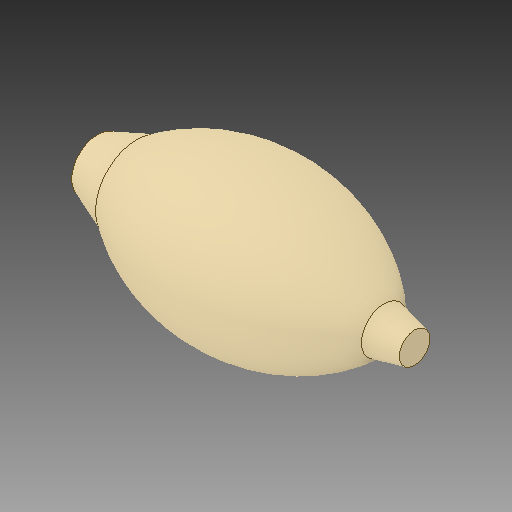
# Autodesk Inventor part: Armbu
Saved by Autodesk Inventor 2019 (Build 230136000, 136)
## iProperties
Created: 2020-04-02
Part Number: Armbu
Material: Generic
Document SubType Name: Modeling
Designer: Jurgen
Density: 1 g/cm^3
Appearance: Beige
Mass: 1875.66 g
Surface Area: 804.648 cm^2
Volume: 1875.66 cm^3
Author: Jurgen
Autodesk Inventor part; units mm, degrees
ref_plane "YZ Plane" through (0, 0, 0) normal (1, 0, 0) x (0, 1, 0)
ref_plane "XZ Plane" through (0, 0, 0) normal (0, 1, 0) x (-1, 0, 0)
ref_plane "XY Plane" through (0, 0, 0) normal (0, 0, 1) x (1, 0, 0)
sketch "Sketch1" plane through (0, 0, 0) normal (0, 0, 1) x (1, 0, 0)
  line L0 (0, 0) -> (-202, 0)
  line L1 (-101, 0) -> (-101, 63.5) construction
  line L2 (-202, 0) -> (-202, 33.5) construction
  line L3 (0, 0) -> (0, 18.5) construction
  arc A0 (0, 18.5) -> (-202, 33.5) centre (-109.7634, -92.0133) ccw
  line L4 (-202, 0) -> (-234, 0)
  line L5 (-234, 0) -> (-234, 21)
  line L6 (-234, 21) -> (-202, 33.5)
  line L7 (0, 0) -> (25, 0)
  line L8 (25, 0) -> (25, 12.5)
  line L9 (0, 18.5) -> (25, 12.5)
  dimension "d0" = 202
  dimension "d1" = 63.5
  dimension "d2" = 33.5
  dimension "d3" = 18.5
  dimension "d4" = 32
  dimension "d5" = 21
  dimension "d6" = 25
  dimension "d7" = 12.5
  constraints: 20 end point, 3 horizontal, 3 point on circle, 3 vertical, 2 perpendicular, 1 centre point, 1 midpoint
  measures "d0" distance of L0.start L0.end
  measures "d1" distance of L1.start L1.end
  measures "d2" distance of L0.end L2.end
  measures "d3" distance of L0.start L3.end
  measures "d4" distance of L0.end L4.end
  measures "d5" distance of L4.end L5.end
  measures "d6" distance of L0.start L7.end
  measures "d7" distance of L7.end L8.end
revolve "Revolution1" add sketch "Sketch1" angle 360 about axis through (0, 0, 0) along (-1, 0, 0)
body "Solid1"
